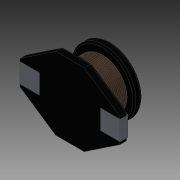
# Autodesk Inventor part: PA6512
Saved by Autodesk Inventor 2013 (Build 170138000, 138)
## iProperties
Created: 2015-07-04
Part Number: PA6512
Material: Ogólny
Document SubType Name: Modeling
Designer: terg
Density: 1 g/cm^3
Author: terg
Autodesk Inventor part; units mm, degrees
ref_plane "YZ Plane" through (0, 0, 0) normal (1, 0, 0) x (0, 1, 0)
ref_plane "XZ Plane" through (0, 0, 0) normal (0, 1, 0) x (-1, 0, 0)
sketch "Szkic1" plane through (0, 0, 0) normal (0, 1, 0) x (-1, 0, 0)
  line L0 (4.625, 0) -> (8.325, 0)
  line L1 (12.95, 3.11) -> (12.95, 6.29)
  line L2 (8.325, 9.4) -> (4.625, 9.4)
  line L3 (0, 6.29) -> (0, 3.11)
  line L4 (0, 6.29) -> (4.625, 9.4)
  line L5 (0, 3.11) -> (4.625, 0)
  line L6 (8.325, 9.4) -> (12.95, 6.29)
  line L7 (8.325, 0) -> (12.95, 3.11)
  point P0 (0, 0)
  point P1 (12.95, 9.4)
  point P2 (12.95, 0)
  point P3 (0, 9.4)
  dimension "d0" = 12.95
  dimension "d1" = 9.4
  dimension "d2" = 3.11
  dimension "d3" = 4.625
  dimension "d4" = 3.11
  dimension "d5" = 4.625
  dimension "d6" = 4.625
  dimension "d7" = 3.11
  dimension "d8" = 4.625
  dimension "d9" = 3.11
  constraints: 16 end point, 8 point on line, 2 parallel, 1 horizontal, 1 perpendicular
  measures "d0" distance of point (0, 9.4) point (12.95, 9.4)
  measures "d1" distance of point (12.95, 9.4) point (12.95, 0)
  measures "d2" distance of L3.start point (0, 9.4)
  measures "d3" distance of L2.end point (0, 9.4)
  measures "d4" distance of L3.end point (0, 0)
  measures "d5" distance of L0.start point (0, 0)
  measures "d6" distance of L2.start point (12.95, 9.4)
  measures "d7" distance of L1.end point (12.95, 9.4)
  measures "d8" distance of L0.end point (12.95, 0)
  measures "d9" distance of L1.start point (12.95, 0)
extrude "Wyciągnięcie proste1" add sketch "Szkic1" along normal blind 1
sketch "Szkic2" plane through (0, 1, 0) normal (0, 1, 0) x (1, 0, 0)
  line L0 (0, -6.29) -> (0, -3.11) projected
  line L1 (-4.625, 0) -> (-8.325, 0) projected
  line L2 (-12.95, -3.11) -> (-12.95, -6.29) projected
  line L3 (-8.325, -9.4) -> (-4.625, -9.4) projected
  circle A0 centre (-6.475, -4.7) radius 4.25
  point P0 (0, 0)
  dimension "d12" = 8.5
  dimension "d13" = 6.475
  dimension "d14" = 6.475
  dimension "d15" = 4.7
  dimension "d16" = 4.7
  constraints: 1 centre point
  measures "d12" diameter of A0
  measures "d13" distance from line of L0 A0.centre
  measures "d14" distance from line of L2 A0.centre
  measures "d15" distance from line of L1 A0.centre
  measures "d16" distance from line of L3 A0.centre
extrude "Wyciągnięcie proste2" add sketch "Szkic2" along normal blind 0.5
sketch "Szkic3" plane through (-6.475, 1.5, 4.7) normal (0, 1, 0) x (1, 0, 0)
  circle A0 centre (0, 0) radius 4.25 projected
  circle A1 centre (0, 0) radius 3
  point P0 (6.475, 4.7)
  dimension "d19" = 6
  constraints: 1 centre point, 1 coincident
  measures "d19" diameter of A1
extrude "Wyciągnięcie proste3" add sketch "Szkic3" along normal blind 2.7 contours A1
sketch "Szkic4" plane through (-6.475, 4.2, 4.7) normal (0, 1, 0) x (1, 0, 0)
  circle A0 centre (0, 0) radius 3 projected
  circle A1 centre (0, 0) radius 4.15
  point P0 (6.475, 4.7)
  dimension "d22" = 8.3
  constraints: 1 centre point, 1 coincident
  measures "d22" diameter of A1
extrude "Wyciągnięcie proste4" add sketch "Szkic4" along normal blind 1 contours A0 | A1
sketch "Szkic5" plane through (0, 0, 0) normal (0, -1, 0) x (1, 0, 0)
  line L0 (-12.95, 6.29) -> (-12.95, 3.11) projected
  line L1 (0, 3.11) -> (0, 6.29) projected
  line L2 (-12.95, 5.97) -> (-10.42, 5.97)
  line L3 (-10.42, 5.97) -> (-10.42, 3.43)
  line L4 (-10.42, 3.43) -> (-12.96, 3.43)
  line L5 (-12.96, 3.43) -> (-12.96, 5.97)
  line L6 (-2.53, 5.97) -> (0, 5.97)
  line L7 (0, 5.97) -> (0, 3.43)
  line L8 (0.01, 3.43) -> (-2.53, 3.43)
  line L9 (-2.53, 3.43) -> (-2.53, 5.97)
  line L10 (-8.325, 0) -> (-4.625, 0) projected
  line L11 (-12.95, 5.97) -> (-12.96, 5.97)
  line L12 (0.01, 3.43) -> (0.01, 5.97)
  line L13 (0.01, 5.97) -> (0, 5.97)
  point P0 (0, 0)
  dimension "d25" = 2.54
  dimension "d26" = 2.54
  dimension "d27" = 0.32
  dimension "d28" = 0.32
  dimension "d29" = 2.54
  dimension "d30" = 2.54
  dimension "d31" = 0.32
  dimension "d36" = 0.01
  dimension "d37" = 0.01
  constraints: 22 end point, 5 parallel, 4 perpendicular, 2 horizontal
  measures "d25" distance of L3.end L4.end
  measures "d26" distance of L2.end L3.end
  measures "d27" distance from line of L0.start L2
  measures "d28" distance from line of L0.end L4
  measures "d29" distance between parallel lines of L8 L6
  measures "d30" distance of L8.start L8.end
  measures "d31" distance from line of L1.start L8
  measures "d36" distance between parallel lines of L0 L5
  measures "d37" distance between parallel lines of L1 L12
extrude "Wyciągnięcie proste5" add sketch "Szkic5" along normal blind 0.01 and the other way blind 1.01
ref_plane "Płaszczyzna konstrukcyjna1" through (-6.475, -0.01, 5.97) normal (1, 0, 0) x (0, 0, -1)
sketch "Szkic6" plane through (-6.475, -0.01, 5.97) normal (1, 0, 0) x (0, 0, -1)
  circle A0 centre (4.37, 1.61) radius 0.1
  line L0 (4.27, 4.21) -> (-1.73, 4.21) projected
  line L1 (-1.73, 1.51) -> (4.27, 1.51) projected
  line L2 (4.27, 1.51) -> (4.27, 4.21) projected
  line L3 (-1.73, 1.51) -> (-1.73, 4.21) projected
  line L4 (1.27, 4.21) -> (1.27, 1.51) construction
  point P0 (5.97, 0.01)
  dimension "d39" = 0.2
  dimension "d40" = 0.1
  dimension "d41" = 0.1
  constraints: 2 end point, 2 midpoint, 1 centre point
  measures "d39" diameter of A0
  measures "d40" distance from line of L2 A0.centre
  measures "d41" distance from line of L1 A0.centre
coil "Zwój1" sketch "Szkic6" operation add axis through (-6.475, 4.2, 4.7) along (0, 1, 0) pitch 0.2005 turns 14.962594 hand right contours A0
sketch "Szkic7" plane through (-6.475, -0.01, 5.97) normal (1, 0, 0) x (0, 0, -1)
  arc A0 (4.27, 1.61) -> (4.37, 1.51) centre (4.37, 1.61) ccw projected
  arc A1 (4.47, 1.61) -> (4.27, 1.61) centre (4.37, 1.61) ccw projected
  arc A2 (4.37, 1.51) -> (4.47, 1.61) centre (4.37, 1.61) ccw projected
  line L0 (4.27, 1.51) -> (4.27, 4.21) projected
  line L1 (-1.73, 1.51) -> (-1.73, 4.21) projected
  line L2 (1.27, 3.9193) -> (1.27, 1.819) construction
  point P0 (5.97, 0.01)
  dimension "d50" = 3
  dimension "d51" = 3
  constraints: 2 end point, 1 parallel
  measures "d50" distance between parallel lines of L0 L2
  measures "d51" distance between parallel lines of L1 L2
coil "Zwój2" sketch "Szkic7" operation add axis through (-6.475, 3.9093, 4.7) along (0, -1, 0) pitch 0.2005 turns 4.987531 hand right
fillet "Zaokrąglenie1" radius 0.2 3 edges at (-10.625, 5.2, 4.7) (-10.625, 4.2, 4.7) (-10.725, 1.5, 4.7)
fillet "Zaokrąglenie2" radius 0.2 10 edges at (-12.95, 1, 3.27) (-12.95, 1, 6.13) (-10.6375, 1, 7.845) (-6.475, 1, 9.4) (-2.3125, 1, 7.845) (-10.6375, 1, 1.555) (-6.475, 1, 0) (-2.3125, 1, 1.555) (0, 1, 3.27) (0, 1, 6.13)
equation "\"d13\" = d14"
equation "\"d15\" = d16"
equation "\"d27\" = d28"
equation "\"d29\" = d26"
equation "\"d30\" = d25"
equation "\"d31\" = d28"
equation "\"d40\" = 0.5 * d39"
equation "\"d41\" = 0.5 * d39"
equation "\"d50\" = d51"
